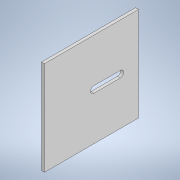
# Autodesk Inventor part: Prototype Panel2
Saved by Autodesk Inventor 2022 (Build 260153000, 153)
## iProperties
Created: 2022-01-20
Part Number: Prototype Panel2
Material: Generic
Document SubType Name: Modeling
Designer: tagaz
Density: 1 g/cm^3
Appearance: Default
Author: tagaz
Autodesk Inventor part; units mm, degrees
ref_plane "YZ Plane" through (0, 0, 0) normal (1, 0, 0) x (0, 1, 0)
ref_plane "XZ Plane" through (0, 0, 0) normal (0, 1, 0) x (-1, 0, 0)
ref_plane "XY Plane" through (0, 0, 0) normal (0, 0, 1) x (1, 0, 0)
sketch "Sketch1" plane through (0, 0, 0) normal (1, 0, 0) x (0, 1, 0)
  line L0 (0, 0) -> (406.4, 0)
  line L1 (406.4, 0) -> (406.4, -406.4)
  line L2 (406.4, -406.4) -> (0, -406.4)
  line L3 (0, -406.4) -> (0, 0)
  dimension "d0" = 406.4
  dimension "d1" = 406.4
  constraints: 8 end point, 2 parallel, 1 horizontal, 1 perpendicular
  measures "d0" distance of L1.end L2.end
  measures "d1" distance of L0.end L1.end
extrude "Extrusion1" add sketch "Sketch1" along normal blind 12.7
sketch "Sketch2" plane through (12.7, 0, 0) normal (1, 0, 0) x (0, 0, -1)
  arc A0 (253.151, 217.4875) -> (253.151, 188.9125) centre (133.35, 203.2) ccw
  arc A1 (278.9512, 188.9125) -> (278.9512, 217.4875) centre (327.7007, 203.2) ccw
  line L0 (0, 406.4) -> (0, 0) projected
  line L1 (406.4, 406.4) -> (0, 406.4) projected
  line L2 (327.7007, 203.2) -> (213.4007, 203.2) construction
  line L3 (327.7007, 217.4875) -> (213.4007, 217.4875)
  line L4 (213.4007, 188.9125) -> (327.7007, 188.9125)
  arc A2 (327.7007, 188.9125) -> (327.7007, 217.4875) centre (327.7007, 203.2) ccw
  arc A3 (213.4007, 217.4875) -> (213.4007, 188.9125) centre (213.4007, 203.2) ccw
  point P0 (270.5507, 203.2)
  dimension "d4" = 241.3
  dimension "d5" = 101.6
  dimension "d6" = 133.35
  dimension "d7" = 12.7
  dimension "d8" = 203.2
  dimension "d9" = 203.2
  dimension "d10" = 114.3
  dimension "d11" = 28.575
  constraints: 8 end point, 8 point on circle, 4 centre point, 4 point on line, 4 tangent, 1 horizontal, 1 midpoint, 1 parallel
  measures "d4" diameter of A0
  measures "d5" diameter of A1
  measures "d6" distance from line of L0 A0.centre
  measures "d7" distance edge to line of A0 L0
  measures "d8" distance from line of L1 L2.start
  measures "d9" distance from line of L1 A0.centre
  measures "d10" distance of L2.start L2.end
  measures "d11" diameter of A3
extrude "Extrusion2" cut sketch "Sketch2" against normal blind 25.4 contours L3 A2 L4 A3
body "Solid1"
